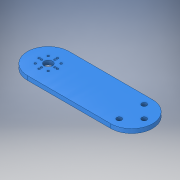
# Autodesk Inventor part: 000.401 - Опорная платформа
Saved by Autodesk Inventor 2019 (Build 230136000, 136)
## iProperties
Created: 2020-03-18
Part Number: 000.401 - Опорная платформа
Material: Пластик АБС
Document SubType Name: Modeling
Designer: Петров Иван
Density: 1.06 g/cm^3
Appearance: Голубой
Author: Петров Иван
Autodesk Inventor part; units mm, degrees
ref_plane "YZ Plane" through (0, 0, 0) normal (1, 0, 0) x (0, 1, 0)
ref_plane "XZ Plane" through (0, 0, 0) normal (0, 1, 0) x (-1, 0, 0)
ref_plane "XY Plane" through (0, 0, 0) normal (0, 0, 1) x (1, 0, 0)
sketch "Эскиз1" plane through (0, 0, 0) normal (0, 1, 0) x (-1, 0, 0)
  circle A0 centre (0, 0) radius 13.8
  circle A1 centre (-8, 0) radius 1.2
  circle A2 centre (0, -8) radius 1.2
  circle A3 centre (8, 0) radius 1.2
  circle A4 centre (0, 8) radius 1.2
  circle A5 centre (-7.7782, 7.7782) radius 1.2813
  circle A6 centre (-11, 0) radius 1.2813
  circle A7 centre (-7.7782, -7.7782) radius 1.2813
  circle A8 centre (0, -11) radius 1.2812
  circle A9 centre (7.7782, -7.7782) radius 1.2812
  circle A10 centre (11, 0) radius 1.2813
  circle A11 centre (7.7782, 7.7782) radius 1.2812
  circle A12 centre (0, 11) radius 1.2812
  circle A13 centre (0, 0) radius 5
  circle A14 centre (0, 0) radius 14
  circle A15 centre (0, 0) radius 1.55
  circle A16 centre (0, 0) radius 1.75
  circle A17 centre (0, 0) radius 25
  dimension "d0" = 50
  constraints: 18 centre point, 1 coincident
  measures "d0" diameter of A17
extrude "Выдавливание1" add sketch "Эскиз1" along normal blind 5 contours A0 | A14 | A17
sketch "Эскиз2" plane through (0, 5, 0) normal (0, 1, 0) x (1, 0, 0)
  line L0 (25, 0) -> (100, 0)
  circle A0 centre (100, 0) radius 25
  line L1 (50, 0) -> (50, -20)
  line L2 (50, 0) -> (50, 20)
  circle A1 centre (0, 0) radius 25 projected
  arc A2 (4.9455, 24.506) -> (95.0545, 24.506) centre (50, 247.5) ccw
  arc A3 (95.0545, -24.506) -> (4.9455, -24.506) centre (50, -247.5) ccw
  line L3 (100, 25) -> (0, 25)
  line L4 (0, -25) -> (100, -25)
  dimension "d3" = 100
  dimension "d4" = 50
  dimension "d5" = 20
  dimension "d6" = 20
  constraints: 15 point on circle, 10 end point, 3 centre point, 3 tangent, 2 vertical, 1 coincident, 1 horizontal, 1 point on line
  measures "d3" distance of point (0, 0) L0.end
  measures "d4" diameter of A0
  measures "d5" distance of L1.start L1.end
  measures "d6" distance of L1.start L2.end
extrude "Выдавливание2" add sketch "Эскиз2" against normal blind 5 contours A1 A2 L2 L0 | L0 L1 A3 A1 | L2 A2 A0 L0 | L0 A0 A3 L1 | A1 L3 A0 A2 | A3 A0 L4 A1 | A0
sketch "Эскиз7" plane through (0, 5, 0) normal (0, 1, 0) x (1, 0, 0)
  line L0 (100, 0) -> (100, 15)
  line L1 (100, 0) -> (100, -15)
  circle A0 centre (100, 15) radius 3
  circle A1 centre (100, -15) radius 3
  line L2 (100, 0) -> (115, 0)
  circle A2 centre (115, 0) radius 3
  point P0 (0, 0)
  dimension "d23" = 15
  dimension "d24" = 15
  dimension "d25" = 6
  dimension "d26" = 6
  dimension "d27" = 15
  dimension "d28" = 6
  constraints: 6 end point, 3 centre point, 3 coincident, 2 vertical, 1 horizontal, 1 other
  measures "d23" distance of L0.start L0.end
  measures "d24" distance of L0.start L1.end
  measures "d25" diameter of A0
  measures "d26" diameter of A1
  measures "d27" distance of L0.start L2.end
  measures "d28" diameter of A2
extrude "Выдавливание7" cut sketch "Эскиз7" against normal blind 10
equation "\"d6\" = d5"
equation "\"d24\" = d23"
equation "\"d26\" = d25"
equation "\"d27\" = d23"
equation "\"d28\" = d25"
